BGC3.1 (Autodesk Fusion 360 design; units mm, degrees)
Autodesk Fusion 360 part; units mm, degrees
sketch "Sketch1" plane through (0, 0, 0) normal (0, 0, 1) x (1, 0, 0)
  line L0 (-25, 25) -> (25, 25) construction
  line L1 (25, 25) -> (25, -25) construction
  line L2 (25, -25) -> (-25, -25) construction
  line L3 (-25, -25) -> (-25, 25) construction
  line L4 (-25, 25) -> (25, -25) construction
  line L5 (25, 25) -> (-25, -25) construction
  line L6 (24, 24) -> (-24, 24) construction
  line L7 (-24, 24) -> (-24, -24) construction
  line L8 (-24, -24) -> (24, -24) construction
  line L9 (24, -24) -> (24, 24) construction
  line L10 (24, 24) -> (-24, -24) construction
  line L11 (-24, 24) -> (24, -24) construction
  circle A0 centre (-22.5, 22.5) radius 1.5
  line L12 (0, 24) -> (0, -24)
  line L13 (-24, 0) -> (24, 0)
  circle A1 centre (-22.5, 22.5) radius 2.5 construction
  line L14 (-25, 0) -> (-25, 22.5)
  line L15 (0, 25) -> (-22.5, 25)
  arc A2 (-22.5, 25) -> (-25, 22.5) centre (-22.5, 22.5) ccw
  circle A3 centre (22.5, 22.5) radius 1.5
  arc A4 (25, 22.5) -> (22.5, 25) centre (22.5, 22.5) ccw
  line L16 (25, 0) -> (25, 22.5)
  line L17 (0, 25) -> (22.5, 25)
  circle A5 centre (-22.5, -22.5) radius 1.5
  arc A6 (-25, -22.5) -> (-22.5, -25) centre (-22.5, -22.5) ccw
  arc A7 (22.5, -25) -> (25, -22.5) centre (22.5, -22.5) ccw
  line L18 (25, 0) -> (25, -22.5)
  line L19 (0, -25) -> (-22.5, -25)
  line L20 (0, -25) -> (22.5, -25)
  line L21 (-25, 0) -> (-25, -22.5)
  circle A8 centre (22.5, -22.5) radius 1.5
  dimension "d1" = 50
  dimension "d2" = 50
  dimension "d3" = 48
  dimension "d4" = 48
  dimension "d5" = 1.5
  constraint horizontal L0
  constraint perpendicular L0 L1
  constraint parallel L0 L2
  constraint parallel L1 L3
  constraint coincident L4 origin
  constraint coincident L5 origin
  constraint horizontal L6
  constraint perpendicular L6 L7
  constraint parallel L6 L8
  constraint parallel L7 L9
  constraint coincident L10 origin
  constraint coincident L11 origin
  constraint tangent L6 A0
  constraint tangent L7 A0
  constraint midpoint L6 L12.start
  constraint midpoint L8 L12.end
  constraint midpoint L7 L13.start
  constraint midpoint L9 L13.end
  constraint concentric A0 A1
  constraint tangent L3 A1
  constraint midpoint L3 L14.start
  constraint coincident L3 L14.end
  constraint coincident A1 L14.end
  constraint midpoint L0 L15.start
  constraint coincident A1 L15.end
  constraint coincident L0 L15.end
  constraint tangent L14 A2
  constraint symmetric A0 L12 A3
  constraint symmetric L12 L14.start L16.start
  constraint symmetric L12 L14.end A4.start
  constraint symmetric L12 L15.start L17.start
  constraint symmetric L12 L15.end A4.end
  constraint symmetric L12 A2 A4
  constraint symmetric A0 L13 A5
  constraint symmetric L13 L14.start L21.start
  constraint symmetric L13 L14.end A6.start
  constraint symmetric L13 L15.start L19.start
  constraint symmetric L13 L15.end A6.end
  constraint symmetric L13 A2 A6
  constraint symmetric L13 A3 A8
  constraint symmetric L13 A4.end A7.start
  constraint symmetric L13 A4.start A7.end
  constraint symmetric L13 A4 A7
  constraint symmetric L13 L16.start L18.start
  measures "d1" distance of L1.end L2.end
  measures "d2" distance of L0.end L1.end
  measures "d3" distance of L7.end L8.end
  measures "d4" distance of L6.end L7.end
  measures "d5" radius of A0
extrude "Extrude1" add sketch "Sketch1" along normal blind 3
sketch "Sketch2" plane through (0, 0, 3) normal (0, 0, 1) x (-1, 0, 0)
  circle A0 centre (22.5, -22.5) radius 1.5
  circle A1 centre (-22.5, -22.5) radius 1.5
  circle A2 centre (-22.5, 22.5) radius 1.5
  circle A3 centre (22.5, 22.5) radius 1.5
  line L0 (-22.5, -25) -> (22.5, -25)
  arc A4 (22.5, -25) -> (25, -22.5) centre (22.5, -22.5) ccw
  line L1 (25, -22.5) -> (25, 22.5)
  arc A5 (25, 22.5) -> (22.5, 25) centre (22.5, 22.5) ccw
  line L2 (22.5, 25) -> (-22.5, 25)
  arc A6 (-22.5, 25) -> (-25, 22.5) centre (-22.5, 22.5) ccw
  line L3 (-25, 22.5) -> (-25, -22.5)
  arc A7 (-25, -22.5) -> (-22.5, -25) centre (-22.5, -22.5) ccw
  line L4 (18, 20) -> (10, 20)
  line L5 (10, 20) -> (10, 27)
  line L6 (10, 27) -> (18, 27)
  line L7 (18, 27) -> (18, 20)
  line L8 (8.1443, 19.89) -> (1.4935, 19.89)
  line L9 (1.4935, 19.89) -> (1.4935, 25)
  line L10 (1.4935, 25) -> (8.1443, 25)
  line L11 (8.1443, 25) -> (8.1443, 19.89)
  line L12 (-6.1327, 6.202) -> (-13.0241, 6.202)
  line L13 (-13.0241, 6.202) -> (-13.0241, 13.2304)
  line L14 (-13.0241, 13.2304) -> (-6.1327, 13.2304)
  line L15 (-6.1327, 13.2304) -> (-6.1327, 6.202)
  line L16 (9.0194, 12.5915) -> (1.9406, 12.5915)
  line L17 (1.9406, 12.5915) -> (1.9406, 3.3668)
  line L18 (1.9406, 3.3668) -> (9.0194, 3.3668)
  line L19 (9.0194, 3.3668) -> (9.0194, 12.5915)
  line L20 (18.1054, 2.8016) -> (12.2514, 2.8016)
  line L21 (12.2514, 2.8016) -> (12.2514, 8.8879)
  line L22 (12.2514, 8.8879) -> (18.1054, 8.8879)
  line L23 (18.1054, 8.8879) -> (18.1054, 2.8016)
  line L24 (23.1634, -18.1139) -> (7.6017, -18.1139)
  line L25 (7.6017, -18.1139) -> (7.6017, -12.2414)
  line L26 (7.6017, -12.2414) -> (23.1634, -12.2414)
  line L27 (23.1634, -12.2414) -> (23.1634, -18.1139)
  line L28 (-1.1153, -18.1139) -> (-17.3248, -18.1139)
  line L29 (-17.3248, -18.1139) -> (-17.3248, -12.2845)
  line L30 (-17.3248, -12.2845) -> (-1.1153, -12.2845)
  line L31 (-1.1153, -12.2845) -> (-1.1153, -18.1139)
  line L32 (17.5, -21) -> (9.5, -21)
  line L33 (9.5, -21) -> (9.5, -29)
  line L34 (9.5, -29) -> (17.5, -29)
  line L35 (17.5, -29) -> (17.5, -21)
  line L36 (-4, -21) -> (-12, -21)
  line L37 (-12, -21) -> (-12, -29)
  line L38 (-12, -29) -> (-4, -29)
  line L39 (-4, -29) -> (-4, -21)
  line L40 (-21.1194, -13.1989) -> (-25, -13.1989)
  line L41 (-25, -13.1989) -> (-25, -6.7401)
  line L42 (-25, -6.7401) -> (-21.1194, -6.7401)
  line L43 (-21.1194, -6.7401) -> (-21.1194, -13.1989)
  line L44 (-17, -0.5) -> (-33, -0.5)
  line L45 (-33, -0.5) -> (-33, 5.5)
  line L46 (-33, 5.5) -> (-17, 5.5)
  line L47 (-17, 5.5) -> (-17, -0.5)
  dimension "d8" = 2
  dimension "d9" = 7
  dimension "d10" = 8
  dimension "d11" = 7
  dimension "d12" = 4
  dimension "d13" = 8
  dimension "d14" = 8
  dimension "d15" = 8
  dimension "d16" = 7.5
  dimension "d17" = 13
  dimension "d18" = 8
  dimension "d19" = 6
  dimension "d20" = 16
  dimension "d21" = 19.5
  constraint horizontal L4
  constraint vertical L5
  constraint horizontal L6
  constraint vertical L7
  constraint horizontal L8
  constraint vertical L9
  constraint horizontal L10
  constraint vertical L11
  constraint coincident L2 L9.end
  constraint horizontal L12
  constraint vertical L13
  constraint horizontal L14
  constraint vertical L15
  constraint horizontal L16
  constraint vertical L17
  constraint horizontal L18
  constraint vertical L19
  constraint horizontal L20
  constraint vertical L21
  constraint horizontal L22
  constraint vertical L23
  constraint horizontal L24
  constraint vertical L25
  constraint horizontal L26
  constraint vertical L27
  constraint horizontal L28
  constraint vertical L29
  constraint horizontal L30
  constraint vertical L31
  constraint horizontal L32
  constraint vertical L33
  constraint horizontal L34
  constraint vertical L35
  constraint horizontal L36
  constraint vertical L37
  constraint horizontal L38
  constraint vertical L39
  constraint collinear L34 L38
  constraint collinear L32 L36
  constraint horizontal L40
  constraint vertical L41
  constraint horizontal L42
  constraint vertical L43
  constraint coincident L3 L41.end
  constraint horizontal L44
  constraint vertical L45
  constraint horizontal L46
  constraint vertical L47
  measures "d8" distance of L2 L6
  measures "d9" distance of L4.start L6.end
  measures "d10" distance of L5.end L6.end
  measures "d11" distance of L1 L7
  measures "d12" distance of L0 L34
  measures "d13" distance of L32.start L34.end
  measures "d14" distance of L33.end L34.end
  measures "d15" distance of L37.end L38.end
  measures "d16" distance of L1 L35
  measures "d17" distance of L3 L37
  measures "d18" distance of L3 L45
  measures "d19" distance of L44.end L45.end
  measures "d20" distance of L45.end L46.end
  measures "d21" distance of L2 L46
extrude "Extrude2" add sketch "Sketch2" along normal blind 8 contours L3 L44 L45 L46 | L3 L44 L46 L47
extrude "Extrude3" add sketch "Sketch2" along normal blind 5 contours L0 L36 L37 L39 | L0 L37 L38 L39 | L0 L32 L33 L35 | L0 L33 L34 L35
extrude "Extrude4" add sketch "Sketch2" along normal blind 3 contours L3 L40 L41 L42 L43 | L2 L8 L9 L10 L11 | L2 L4 L5 L7 | L2 L5 L6 L7
extrude "Extrude5" add sketch "Sketch2" along normal blind 2 contours L16 L17 L18 L19
extrude "Extrude6" add sketch "Sketch2" along normal blind 1.5 contours L12 L13 L14 L15 | L20 L21 L22 L23 | L24 L25 L26 L27 | L28 L29 L30 L31
sketch "Sketch3" plane through (0, 0, 3) normal (0, 0, 1) x (-1, 0, 0)
  line L0 (-1.1153, -12.2845) -> (-1.1153, -18.1139)
  line L1 (-1.1153, -18.1139) -> (-17.3248, -18.1139)
  line L2 (-17.3248, -18.1139) -> (-17.3248, -12.2845)
  line L3 (-17.3248, -12.2845) -> (-1.1153, -12.2845)
  line L4 (-6.1327, 13.2304) -> (-6.1327, 6.202)
  line L5 (-6.1327, 6.202) -> (-13.0241, 6.202)
  line L6 (-13.0241, 6.202) -> (-13.0241, 13.2304)
  line L7 (-13.0241, 13.2304) -> (-6.1327, 13.2304)
  line L8 (23.1634, -12.2414) -> (23.1634, -18.1139)
  line L9 (23.1634, -18.1139) -> (7.6017, -18.1139)
  line L10 (7.6017, -18.1139) -> (7.6017, -12.2414)
  line L11 (7.6017, -12.2414) -> (23.1634, -12.2414)
  line L12 (18.1054, 8.8879) -> (18.1054, 2.8016)
  line L13 (18.1054, 2.8016) -> (12.2514, 2.8016)
  line L14 (12.2514, 2.8016) -> (12.2514, 8.8879)
  line L15 (12.2514, 8.8879) -> (18.1054, 8.8879)
  line L16 (9.0194, 3.3668) -> (1.9406, 3.3668)
  line L17 (1.9406, 3.3668) -> (1.9406, 12.5915)
  line L18 (1.9406, 12.5915) -> (9.0194, 12.5915)
  line L19 (9.0194, 12.5915) -> (9.0194, 3.3668)
  line L20 (-21.1194, -13.1989) -> (-25, -13.1989)
  line L21 (-25, -13.1989) -> (-25, -22.5)
  arc A0 (-25, -22.5) -> (-22.5, -25) centre (-22.5, -22.5) ccw
  line L22 (-22.5, -25) -> (-12, -25)
  line L23 (-12, -25) -> (-12, -21)
  line L24 (-12, -21) -> (-4, -21)
  line L25 (-4, -21) -> (-4, -25)
  line L26 (-4, -25) -> (9.5, -25)
  line L27 (9.5, -25) -> (9.5, -21)
  line L28 (9.5, -21) -> (17.5, -21)
  line L29 (17.5, -21) -> (17.5, -25)
  line L30 (17.5, -25) -> (22.5, -25)
  arc A1 (22.5, -25) -> (25, -22.5) centre (22.5, -22.5) ccw
  line L31 (25, -22.5) -> (25, 22.5)
  arc A2 (25, 22.5) -> (22.5, 25) centre (22.5, 22.5) ccw
  line L32 (22.5, 25) -> (18, 25)
  line L33 (18, 25) -> (18, 20)
  line L34 (18, 20) -> (10, 20)
  line L35 (10, 20) -> (10, 25)
  line L36 (10, 25) -> (8.1443, 25)
  line L37 (8.1443, 25) -> (8.1443, 19.89)
  line L38 (8.1443, 19.89) -> (1.4935, 19.89)
  line L39 (1.4935, 19.89) -> (1.4935, 25)
  line L40 (1.4935, 25) -> (-22.5, 25)
  arc A3 (-22.5, 25) -> (-25, 22.5) centre (-22.5, 22.5) ccw
  line L41 (-25, 22.5) -> (-25, 5.5)
  line L42 (-25, 5.5) -> (-17, 5.5)
  line L43 (-17, 5.5) -> (-17, -0.5)
  line L44 (-17, -0.5) -> (-25, -0.5)
  line L45 (-25, -0.5) -> (-25, -6.7401)
  line L46 (-25, -6.7401) -> (-21.1194, -6.7401)
  line L47 (-21.1194, -6.7401) -> (-21.1194, -13.1989)
  circle A4 centre (22.5, -22.5) radius 1.5
  circle A5 centre (-22.5, -22.5) radius 1.5
  circle A6 centre (-22.5, 22.5) radius 1.5
  circle A7 centre (22.5, 22.5) radius 1.5
  line L48 (4.6554, 14.7653) -> (3.1888, 14.7653)
  line L49 (3.1888, 14.7653) -> (3.1888, 15.6382)
  line L50 (3.1888, 15.6382) -> (4.6554, 15.6382)
  line L51 (4.6554, 15.6382) -> (4.6554, 14.7653)
  line L52 (4.6554, 16.2319) -> (3.1888, 16.2319)
  line L53 (3.1888, 16.2319) -> (3.1888, 17.2096)
  line L54 (3.1888, 17.2096) -> (4.6554, 17.2096)
  line L55 (4.6554, 17.2096) -> (4.6554, 16.2319)
  constraint horizontal L48
  constraint vertical L49
  constraint horizontal L50
  constraint vertical L51
  constraint horizontal L52
  constraint vertical L53
  constraint horizontal L54
  constraint vertical L55
extrude "Extrude7" add sketch "Sketch3" along normal blind 0.1 contours L48 L49 L50 L51 | L52 L53 L54 L55
equation "d15 = d14"
